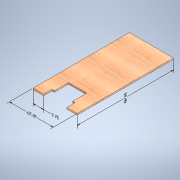
# Autodesk Inventor part: 2020 Wood BaseV04
Saved by Autodesk Inventor 2020.2 (Build 242310000, 310)
## iProperties
Created: 2020-01-12
Part Number: 2020 Wood BaseV04
Material: Wood (Birch)
Document SubType Name: Modeling
Designer: robst
Density: 0.55 g/cm^3
Appearance: Birch - Natural Polished
Author: robst
Autodesk Inventor part; units mm, degrees
ref_plane "YZ Plane" through (0, 0, 0) normal (1, 0, 0) x (0, 1, 0)
ref_plane "XZ Plane" through (0, 0, 0) normal (0, 1, 0) x (-1, 0, 0)
ref_plane "XY Plane" through (0, 0, 0) normal (0, 0, 1) x (1, 0, 0)
sketch "Sketch1" plane through (0, 0, 0) normal (0, 1, 0) x (-1, 0, 0)
  line L0 (200.025, 436.88) -> (-200.025, 436.88)
  line L1 (-200.025, 436.88) -> (-200.025, -436.88)
  line L2 (-200.025, -436.88) -> (200.025, -436.88)
  line L3 (200.025, -436.88) -> (200.025, 436.88)
  line L4 (200.025, 436.88) -> (-200.025, -436.88) construction
  line L5 (-200.025, 436.88) -> (200.025, -436.88) construction
  point P0 (0, 0)
  dimension "d0" = 400.05
  dimension "d1" = 873.76
  constraints: 12 end point, 2 midpoint, 2 parallel, 1 horizontal, 1 perpendicular
  measures "d0" distance of L0.start L0.end
  measures "d1" distance of L1.end L0.end
extrude "Extrusion1" add sketch "Sketch1" along normal blind 12.7
sketch "Sketch4" plane through (0, 12.7, 0) normal (0, 1, 0) x (1, 0, 0)
  line L0 (-82.55, -436.88) -> (82.55, -436.88)
  line L1 (82.55, -436.88) -> (82.55, -233.68)
  line L2 (82.55, -233.68) -> (-82.55, -233.68)
  line L3 (-82.55, -233.68) -> (-82.55, -436.88)
  line L4 (-82.55, -436.88) -> (82.55, -233.68) construction
  line L5 (82.55, -436.88) -> (-82.55, -233.68) construction
  line L6 (-200.025, -436.88) -> (200.025, -436.88) projected
  line L7 (-200.025, 436.88) -> (-200.025, -436.88) projected
  line L8 (200.025, -436.88) -> (200.025, 436.88) projected
  point P0 (0, 0)
  point P1 (0, -335.28)
  dimension "d11" = 0
  dimension "d12" = 165.1
  dimension "d13" = 203.2
  dimension "d19" = 117.475
  dimension "d20" = 117.475
  constraints: 12 end point, 2 midpoint, 2 parallel, 1 collinear, 1 horizontal, 1 perpendicular
  measures "d11" horizontal distance of point (0, 0) point (0, -335.28)
  measures "d12" distance of L0.start L0.end
  measures "d13" distance of L0.end L1.end
  measures "d19" distance between parallel lines of L3 L7
  measures "d20" distance between parallel lines of L8 L1
extrude "Extrusion2" cut sketch "Sketch4" against normal through all
sketch "Sketch6" plane through (0, 12.7, 0) normal (0, 1, 0) x (1, 0, 0)
  line L0 (0, 0) -> (0, -436.88) construction
  line L1 (-104.775, -360.68) -> (104.775, -360.68)
  line L2 (104.775, -360.68) -> (104.775, -436.88)
  line L3 (104.775, -436.88) -> (-104.775, -436.88)
  line L4 (-104.775, -436.88) -> (-104.775, -360.68)
  line L5 (-104.775, -360.68) -> (104.775, -436.88) construction
  line L6 (104.775, -360.68) -> (-104.775, -436.88) construction
  line L7 (-200.025, -436.88) -> (-82.55, -436.88) projected
  point P0 (0, -398.78)
  dimension "d24" = 209.55
  dimension "d25" = 76.2
  constraints: 14 end point, 2 midpoint, 2 parallel, 2 perpendicular, 1 collinear, 1 point on line, 1 vertical
  measures "d24" distance of L1.start L1.end
  measures "d25" distance of L1.end L2.end
extrude "Extrusion4" cut sketch "Sketch6" against normal through all
body "Solid1"
